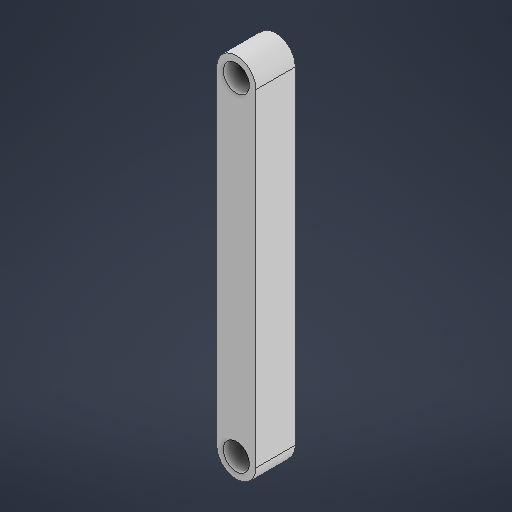
# Autodesk Inventor part: 轴
Saved by Autodesk Inventor 2025 (Build 290162000, 162)
## iProperties
Created: 2026-04-17
Part Number: 轴
Material: 常规
Document SubType Name: Modeling
Designer: XH
Density: 1 g/cm^3
Appearance: 默认
Author: XH
Autodesk Inventor part; units mm, degrees
ref_plane "YZ Plane" through (0, 0, 0) normal (1, 0, 0) x (0, 1, 0)
ref_plane "XZ Plane" through (0, 0, 0) normal (0, 1, 0) x (-1, 0, 0)
ref_plane "XY Plane" through (0, 0, 0) normal (0, 0, 1) x (1, 0, 0)
sketch "草图1" plane through (0, 0, 0) normal (0, 0, 1) x (1, 0, 0)
  line L0 (0, 0) -> (0, 25) construction
  line L1 (1.5, 0) -> (1.5, 25)
  line L2 (-1.5, 25) -> (-1.5, 0)
  arc A0 (-1.5, 0) -> (1.5, 0) centre (0, 0) ccw
  arc A1 (1.5, 25) -> (-1.5, 25) centre (0, 25) ccw
  circle A2 centre (0, 25) radius 1
  circle A3 centre (0, 0) radius 1
  point P0 (0, 12.5)
  dimension "d0" = 2
  dimension "d1" = 1.5
  dimension "d2" = 2
  dimension "d5" = 25
  constraints: 8 end point, 4 centre point, 4 point on circle, 4 tangent, 2 coincident, 1 midpoint, 1 parallel, 1 vertical
  measures "d0" diameter of A2
  measures "d1" radius of A1
  measures "d2" diameter of A3
  measures "d5" distance of L0.end L0.start
extrude "拉伸1" add sketch "草图1" along normal blind 3
